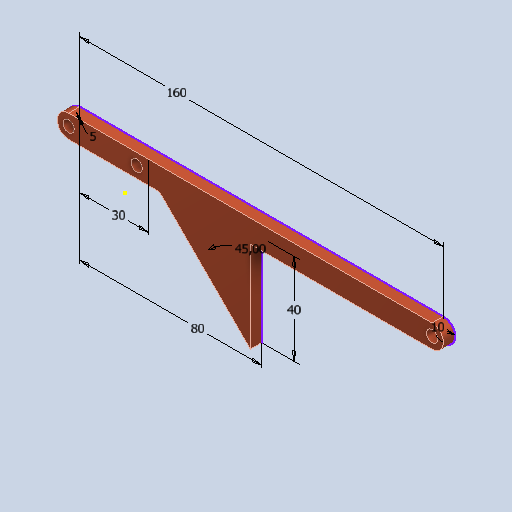
# Autodesk Inventor part: Part1
Saved by Autodesk Inventor 2022 (Build 260153000, 153)
## iProperties
Created: 2022-03-14
Part Number: Part1
Material: Copper, Alloy
Document SubType Name: Modeling
Designer: br4ch
Density: 8.92 g/cm^3
Appearance: Copper - Satin
Mass: 107.916 g
Surface Area: 71.1481 cm^2
Volume: 12.0982 cm^3
Author: br4ch
Autodesk Inventor part; units mm, degrees
ref_plane "YZ Plane" through (0, 0, 0) normal (1, 0, 0) x (0, 1, 0)
ref_plane "XZ Plane" through (0, 0, 0) normal (0, 1, 0) x (-1, 0, 0)
ref_plane "XY Plane" through (0, 0, 0) normal (0, 0, 1) x (1, 0, 0)
sketch "Sketch1" plane through (0, 0, 0) normal (0, 0, 1) x (1, 0, 0)
  line L0 (-20, 17.9339) -> (140, 17.9339) construction
  line L1 (-20, 12.9339) -> (140, 12.9339)
  line L2 (140, 22.9339) -> (-20, 22.9339)
  arc A0 (-20, 22.9339) -> (-20, 12.9339) centre (-20, 17.9339) ccw
  arc A1 (140, 12.9339) -> (140, 22.9339) centre (140, 17.9339) ccw
  circle A2 centre (-20, 17.9339) radius 2.5
  circle A3 centre (140, 17.9339) radius 2.5
  circle A4 centre (10, 17.9339) radius 2.5
  line L3 (60, 12.9339) -> (60, -27.0661)
  line L4 (60, -27.0661) -> (20, 12.9339)
  point P0 (0, 0)
  point P1 (60, 17.9339)
  dimension "d0" = 10
  dimension "d1" = 5
  dimension "d2" = 160
  dimension "d7" = 30
  dimension "d10" = 45
  dimension "d11" = 40
  dimension "d12" = 80
  constraints: 12 end point, 5 centre point, 4 point on circle, 4 tangent, 2 coincident, 2 equal radius, 2 midpoint, 2 point on line, 1 horizontal, 1 parallel, 1 perpendicular
  measures "d0" diameter of A1
  measures "d1" diameter of A2
  measures "d2" distance of L0.end L0.start
  measures "d7" distance of A4.centre L0.start
  measures "d10" angle of L3 L4
  measures "d11" distance of L3.start L3.end
  measures "d12" distance from line of L3 L0.start
extrude "Extrusion1" add sketch "Sketch1" along normal blind 5 contours A0 L2 A1 L1 | A3 | A4
extrude "Extrusion3" cut sketch "Sketch1" along normal up to surface (5 mm away) contours A3 | A4
extrude "Extrusion4" add sketch "Sketch1" along normal up to surface (5 mm away) contours L1 L3 L4
body "Solid1"
